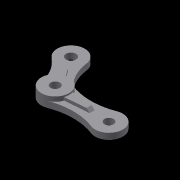
# Autodesk Inventor part: ElbowSubConnectorRight
Saved by Autodesk Inventor 2015 (Build 190159000, 159)
## iProperties
RuleStatus: InUse
Created: 2014-09-28
Part Number: ElbowSubConnectorRight
Material: Generic
Document SubType Name: Modeling
Designer: Inventor
Mass: 5.13678 g
Surface Area: 34.1001 cm^2
Volume: 5.13678 cm^3
Density: 1 g/cm^3
Appearance: Default
BeforeDocSave0: UpdateBoundingBox
CX: 67.00 mm
CY: 42.25 mm
CZ: 7.00 mm
Author: Inventor
Autodesk Inventor part; units mm, degrees
ref_plane "YZ Plane" through (0, 0, 0) normal (1, 0, 0) x (0, 1, 0)
ref_plane "XZ Plane" through (0, 0, 0) normal (0, 1, 0) x (-1, 0, 0)
ref_plane "XY Plane" through (0, 0, 0) normal (0, 0, 1) x (1, 0, 0)
sketch "Base" plane through (0, 0, 0) normal (0, 0, 1) x (1, 0, 0)
  line L0 (-54.6, 0) -> (19.6, 0) construction
  circle A0 centre (0, 0) radius 9
  line L1 (0, 0) -> (-35, 0) construction
  circle A1 centre (-35, 0) radius 9
  arc A2 (-31.7857, 8.4064) -> (-3.2143, 8.4064) centre (-17.5, 45.7684) ccw
  arc A3 (-3.2143, -8.4064) -> (-31.7857, -8.4064) centre (-17.5, -45.7684) ccw
  dimension "d0" = 18
  dimension "d1" = 35
  dimension "d2" = 18
  dimension "d3" = 40
  constraints: 8 point on circle, 4 centre point, 4 tangent, 2 coincident, 2 end point, 1 equal radius, 1 point on line
  measures "d0" diameter of A0
  measures "d1" distance of L1.start L1.end
  measures "d2" diameter of A1
  measures "d3" radius of A2
extrude "BaseFeature" add sketch "Base" along normal blind 4
sketch "Sketch2" plane through (0, 0, 4) normal (0, 0, 1) x (1, 0, 0)
  arc A0 (-31.7857, 8.4064) -> (-31.7857, -8.4064) centre (-35, 0) ccw projected
  arc A1 (-3.2143, -8.4064) -> (-3.2143, 8.4064) centre (0, 0) ccw projected
hole "BaseHolesFeature" at (-35, 0, 4) at (0, 0, 4) direction (0, 0, -1) diameter 6 end through all
sketch "Extension" plane through (0, 0, 4) normal (0, 0, 1) x (1, 0, 0)
  arc A0 (-31.7857, 8.4064) -> (-31.7857, -8.4064) centre (-35, 0) ccw construction
  line L0 (-35, 0) -> (-49, -24.2487) construction
  line L1 (-90.0286, 0) -> (25.5048, 0) construction
  circle A1 centre (-49, -24.2487) radius 9
  arc A2 (-54.6593, -17.2507) -> (-43.8901, 1.4021) centre (-73.5238, 6.0759) ccw
  arc A3 (-31.7857, -8.4064) -> (-40.0784, -25.4338) centre (-10.3396, -29.3841) ccw
  arc A4 (-43.8901, 1.4021) -> (-31.7857, -8.4064) centre (-35, 0) ccw
  dimension "d13" = 120
  dimension "d14" = 28
  dimension "d24" = 18
  dimension "d29" = 30
  constraints: 9 point on circle, 4 centre point, 4 tangent, 2 end point, 1 coincident, 1 equal radius
  measures "d13" angle of L0 L1
  measures "d14" distance of L0.start L0.end
  measures "d24" diameter of A1
  measures "d29" radius of A2
extrude "ExtensionFeature" add sketch "Extension" against normal up to surface (4 mm away)
sketch "ExtensionHole" plane through (0, 0, 0) normal (0, 0, -1) x (-1, 0, 0)
  arc A0 (40.0784, -25.4338) -> (54.6593, -17.2507) centre (49, -24.2487) ccw projected
hole "ExtensionHoleFeature" at (-49, -24.2487, 0) direction (0, 0, 1) diameter 6.5 end through all
sketch "MiddleRaise" plane through (0, 0, 4) normal (0, 0, 1) x (1, 0, 0)
  circle A0 centre (-35, 0) radius 3 projected
  circle A1 centre (-35, 0) radius 9
  point P0 (-31.7857, 8.4064)
  constraints: 1 coincident, 3 other
extrude "MiddleRaiseFeature" add sketch "MiddleRaise" along normal blind 3
sketch "TopRidges" plane through (0, 0, 4) normal (0, 0, 1) x (1, 0, 0)
  arc A0 (-54.6593, -17.2507) -> (-40.0784, -25.4338) centre (-49, -24.2487) ccw construction
  arc A1 (-3.2143, -8.4064) -> (-3.2143, 8.4064) centre (0, 0) ccw construction
  arc A2 (-43.8901, 1.4021) -> (-31.7857, -8.4064) centre (-35, 0) ccw construction
  arc A3 (-31.7857, -8.4064) -> (-31.7857, 8.4064) centre (-35, 0) ccw construction
  line L0 (-35, 0) -> (-49, -24.2487) construction
  line L1 (-40.5981, -3.6962) -> (-35.4019, -6.6962)
  line L2 (-35.4019, -6.6962) -> (-42.201, -15.4724)
  line L3 (-42.201, -15.4724) -> (-44.799, -13.9724)
  line L4 (-44.799, -13.9724) -> (-40.5981, -3.6962)
  arc A4 (-40.0784, -25.4338) -> (-54.6593, -17.2507) centre (-49, -24.2487) ccw construction
  line L5 (-35, 0) -> (-11, 0) construction
  arc A5 (-3.2143, 8.4064) -> (-3.2143, -8.4064) centre (0, 0) ccw construction
  line L6 (-29, 3) -> (-29, -3)
  line L7 (-29, -3) -> (-10.8759, -1.5)
  line L8 (-10.8759, -1.5) -> (-11.1241, 1.5)
  line L9 (-11.1241, 1.5) -> (-29, 3)
  point P0 (-43.5, -14.7224)
  point P1 (-38, -5.1962)
  point P2 (-29, 0)
  dimension "d30" = 3
  dimension "d31" = 6
  dimension "d37" = 6
  dimension "d39" = 11
  dimension "d40" = 11
  dimension "d41" = 6
  dimension "d42" = 6
  dimension "d43" = 3
  constraints: 20 end point, 4 midpoint, 4 point on circle, 3 concentric, 3 perpendicular, 3 point on line, 2 centre point, 1 horizontal, 1 vertical
  measures "d30" distance of L2.end L3.end
  measures "d31" distance of L1.start L1.end
  measures "d37" distance from line of A2.centre L1
  measures "d39" distance from line of L3 A4.centre
  measures "d40" distance of L5.end A5.centre
  measures "d41" distance of point (-29, 0) A2.centre
  measures "d42" distance of L6.start L6.end
  measures "d43" vertical distance of L7.end L8.end
extrude "TopRidgesFeature" add sketch "TopRidges" along normal blind 2
chamfer "TopRidgeChamfersFeature" distance 2 angle 45 2 edges at (-43.5, -14.7224, 6) (-11, 0, 6)
mirror "RightMirror" about plane through (0, 0, 0) normal (0, 1, 0) remove original yes
equation "\"d41\" = d37"
equation "\"d42\" = d31"
equation "\"d43\" = d30"
